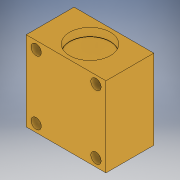
# Autodesk Inventor part: brassbushing2
Saved by Autodesk Inventor 2018 (Build 220112000, 112)
## iProperties
Created: 2019-03-13
Part Number: brassbushing2
Material: Brass, Soft Yellow
Document SubType Name: Modeling
Designer: Admin
Density: 8.47 g/cm^3
Appearance: Brass - Satin
Mass: 52.4793 g
Surface Area: 42.2353 cm^2
Volume: 6.1959 cm^3
Author: Admin
Autodesk Inventor part; units mm, degrees
ref_plane "YZ Plane" through (0, 0, 0) normal (1, 0, 0) x (0, 1, 0)
ref_plane "XZ Plane" through (0, 0, 0) normal (0, 1, 0) x (-1, 0, 0)
ref_plane "XY Plane" through (0, 0, 0) normal (0, 0, 1) x (1, 0, 0)
sketch "Sketch1" plane through (0, 0, 0) normal (0, 1, 0) x (-1, 0, 0)
  circle A0 centre (0, 0) radius 7.62
  line L0 (12.7, 7.62) -> (-12.7, 7.62)
  line L1 (-12.7, 7.62) -> (-12.7, -7.62)
  line L2 (-12.7, -7.62) -> (12.7, -7.62)
  line L3 (12.7, -7.62) -> (12.7, 7.62)
  line L4 (12.7, 7.62) -> (-12.7, -7.62) construction
  line L5 (-12.7, 7.62) -> (12.7, -7.62) construction
  line L6 (12.7, 7.62) -> (38.1, 7.62) construction
  dimension "d0" = 15.24
  dimension "d27" = 25.4
  dimension "d28" = 180
  dimension "d29" = 15.24
  constraints: 14 end point, 2 horizontal, 2 midpoint, 2 parallel, 1 centre point, 1 coincident, 1 collinear, 1 perpendicular
  measures "d0" diameter of A0
  measures "d27" distance of L0.start L0.end
  measures "d28" angle of L0 L6
  measures "d29" distance of L1.end L0.end
extrude "Extrusion1" add sketch "Sketch1" along normal mid plane 25.4
sketch "Sketch2" plane through (0, 12.7, 0) normal (0, 1, 0) x (1, 0, 0)
  circle A0 centre (0, 0) radius 3.175
  dimension "d3" = 6.35
  constraints: 1 centre point, 1 coincident
  measures "d3" diameter of A0
hole "Hole1" at (0, 12.7, 0) direction (0, -1, 0) diameter 10.4648 depth 24.7904 tip angle 118
sketch "Sketch3" plane through (0, 12.7, 0) normal (0, 1, 0) x (1, 0, 0)
  circle A0 centre (0, 0) radius 6.3627
  dimension "d6" = 12.7254
  constraints: 1 centre point, 1 coincident
  measures "d6" diameter of A0
extrude "Extrusion3" cut sketch "Sketch3" against normal blind 11.684
sketch "Sketch4" plane through (0, -12.7, 0) normal (0, -1, 0) x (1, 0, 0)
  circle A0 centre (0, 0) radius 6.3627
  dimension "d9" = 12.7254
  constraints: 1 centre point, 1 coincident
  measures "d9" diameter of A0
extrude "Extrusion4" cut sketch "Sketch4" against normal blind 11.684
sketch "Sketch5" plane through (0, 12.7, 0) normal (0, 1, 0) x (1, 0, 0)
  circle A0 centre (0, 0) radius 6.477
  dimension "d13" = 12.954
  constraints: 1 centre point, 1 coincident
  measures "d13" diameter of A0
extrude "Extrusion5" cut sketch "Sketch5" against normal blind 2.54
sketch "Sketch6" plane through (0, -12.7, 0) normal (0, -1, 0) x (1, 0, 0)
  circle A0 centre (0, 0) radius 6.477
  dimension "d16" = 12.954
  constraints: 1 centre point, 1 coincident
  measures "d16" diameter of A0
extrude "Extrusion6" cut sketch "Sketch6" against normal blind 2.54
sketch "Sketch7" plane through (-12.7, 12.7, 7.62) normal (0, 0, 1) x (1, 0, 0)
  line L0 (3.175, -2.54) -> (22.225, -2.54) construction
  line L1 (22.225, -2.54) -> (22.225, -22.86) construction
  line L2 (22.225, -22.86) -> (3.175, -22.86) construction
  line L3 (3.175, -22.86) -> (3.175, -2.54) construction
  line L4 (3.175, -2.54) -> (22.225, -22.86) construction
  line L5 (22.225, -2.54) -> (3.175, -22.86) construction
  point P0 (12.7, -12.7)
  dimension "d30" = 19.05
  dimension "d31" = 20.32
  constraints: 12 end point, 4 coincident, 2 midpoint, 2 parallel, 1 horizontal, 1 perpendicular
  measures "d30" distance of L1.end L2.end
  measures "d31" distance of L0.end L1.end
hole "Hole2" at (9.525, 10.16, 7.62) at (9.525, -10.16, 7.62) at (-9.525, -10.16, 7.62) at (-9.525, 10.16, 7.62) direction (0, 0, -1) diameter 3.2766 end through all clearance for "Flat Head Machine Screw (82)" size "#4" standard "Ansi Unified Screw Threads"
body "Solid1"
